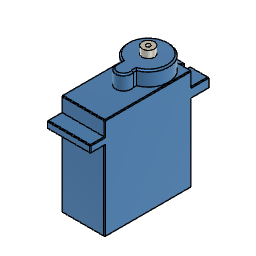
Servo Motor (Autodesk Fusion 360 design; units mm, degrees)
Autodesk Fusion 360 part; units mm, degrees
note: some values were not read from the file. Chosen so that the rebuilt part matches the saved one: a direction.
sketch "Sketch1" plane through (0, 0, 0) normal (1, 0, 0) x (0, 1, 0)
  line L0 (0, 0) -> (60, 0)
  line L1 (60, 0) -> (60, 70)
  line L2 (60, 70) -> (0, 70)
  line L3 (0, 70) -> (0, 0)
  line L4 (0, 50) -> (60, 50)
  dimension "d1" = 60
  dimension "d2" = 70
  constraint horizontal L0
  constraint vertical L1
  constraint horizontal L2
  constraint vertical L3
  constraint coincident L0.start L3.end
  constraint coincident L3 L4.start
  constraint perpendicular L3 L4
  constraint coincident L1 L4.end
  measures "d1" distance of L1.end L2.end
  measures "d2" vertical distance of L0.start L1.end
extrude "Extrude1" add sketch "Sketch1" along normal blind 30 makes body 1
sketch "Sketch2" plane through (0, 0, 70) normal (0, 0, 1) x (-1, 0, 0)
  line L0 (0, -60) -> (0, 0)
  line L1 (0, 0) -> (-30, 0)
  line L2 (-30, 0) -> (-30, -60)
  line L3 (-30, -60) -> (0, -60)
  circle A0 centre (-15, -45) radius 4.4943
  circle A1 centre (-15, -45) radius 1.0141
  line L4 (-10.0834, -31.5246) -> (-10.0834, -25)
  line L5 (-19.9166, -31.5246) -> (-19.9166, -25)
  arc A2 (-10.0834, -25) -> (-19.9166, -25) centre (-15, -25) ccw
  arc A3 (-19.9166, -31.5246) -> (-10.0834, -31.5246) centre (-15, -45) ccw
  dimension "d5" = 28.6886
  dimension "d6" = 8.9885
  dimension "d7" = 2.0283
  dimension "d8" = 9.8331
  constraint concentric A0 A3
  constraint concentric A0 A1
  constraint parallel L0 L4
  constraint parallel L4 L5
  constraint tangent L5 A2
  measures "d5" diameter of A3
  measures "d6" diameter of A0
  measures "d7" diameter of A1
  measures "d8" distance of L4.end L5.end
extrude "Extrude3" add sketch "Sketch2" along normal blind 15 contours A0 bodies 1
sketch "Sketch3" plane through (0, 60, 0) normal (0, 1, 0) x (-1, 0, 0)
  line L0 (0, 0) -> (0, 70)
  line L1 (0, 70) -> (-30, 70)
  line L2 (-30, 70) -> (-30, 0)
  line L3 (-30, 0) -> (0, 0)
  line L4 (-30, 60) -> (0, 60)
  line L5 (0, 60) -> (0, 53.1514)
  line L6 (0, 53.1514) -> (-30, 53.1514)
  line L7 (-30, 53.1514) -> (-30, 60)
  constraint horizontal L4
  constraint vertical L5
  constraint horizontal L6
  constraint vertical L7
  constraint coincident L0 L5.end
  constraint coincident L2 L4.start
extrude "Extrude4" add sketch "Sketch3" along normal blind 12 contours L0 L2 L4 L5 L6 L7 bodies 1
sketch "Sketch4" plane through (0, 0, 60) normal (0, 0, 1) x (-1, 0, 0)
  line L0 (0, -60) -> (-30, -60)
  line L1 (-30, -60) -> (-30, -72)
  line L2 (-30, -72) -> (0, -72)
  line L3 (0, -72) -> (0, -60)
  line L4 (-15, -72) -> (-17, -72)
  line L5 (-15, -72) -> (-13, -72)
  line L6 (-13, -72) -> (-13, -70)
  line L7 (-17, -72) -> (-17, -70)
  arc A0 (-13, -70) -> (-17, -70) centre (-15, -67) ccw
  dimension "d16" = 7.2111
  constraint midpoint L2 L4.start
  constraint coincident L2 L4.end
  constraint parallel L2 L4
  constraint coincident L2 L5.end
  constraint perpendicular L2 L6
  constraint perpendicular L2 L7
  measures "d16" diameter of A0
extrude "Extrude5" cut sketch "Sketch4" against normal through all contours L2 L4 L5 L6 L7 A0 bodies 1
chamfer "Chamfer2" distance 0.5 angle 45 7 edges at (15, 63.3944, 60) (0, 66, 60) (30, 66, 60) (23.5, 72, 60) (6.5, 72, 60) (6.5, 72, 53.1514) (23.5, 72, 53.1514) on bodies 1
chamfer "Chamfer3" distance 0.5 angle 45 7 edges at (0, 65.75, 53.1514) (30, 65.75, 53.1514) (15, 63.3944, 53.1514) (17, 70.75, 53.1514) (13, 70.75, 53.1514) (13, 71.0427, 60) (17, 71.0427, 60) on bodies 1
sketch "Sketch5" plane through (0, 0, 0) normal (0, -1, 0) x (1, 0, 0)
  line L0 (0, 70) -> (0, 0)
  line L1 (0, 0) -> (30, 0)
  line L2 (30, 0) -> (30, 70)
  line L3 (30, 70) -> (0, 70)
  line L4 (0, 60) -> (30, 60)
  line L5 (30, 60) -> (30, 55)
  line L6 (30, 55) -> (0, 55)
  line L7 (0, 55) -> (0, 60)
  constraint horizontal L4
  constraint vertical L5
  constraint horizontal L6
  constraint vertical L7
  constraint coincident L2 L5.end
  constraint coincident L0 L4.start
extrude "Extrude6" add sketch "Sketch5" along normal blind 10 contours L0 L2 L4 L5 L6 L7 bodies 1
chamfer "Chamfer4" distance 0.5 angle 45 8 edges at (30, 30, 70) (30, 60, 26.8257) (30, 0, 27.5) (30, -5, 55) (30, -5, 60) (30, 60, 64.75) (30, 0, 65) (30, 30, 0) on bodies 1
chamfer "Chamfer5" distance 0.5 angle 45 14 edges at (0, 30, 70) (0, 60, 64.75) (0, 60, 26.8257) (0, 0, 65) (0, 0, 27.5) (0, -5, 55) (0, -5, 60) (14.75, -10, 55) (14.75, -10, 60) (30, -10, 57.5) (0, -10, 57.5) (0, 30, 0) (14.75, 0, 0) (29.5, 0, 27.5) on bodies 1
chamfer "Chamfer6" distance 0.5 angle 45 2 edges at (15, 60, 70) (15, 0, 70) on bodies 1
chamfer "Chamfer7" distance 0.5 angle 45 1 edges at (15, 60, 0) on bodies 1
delete_face "DeleteFace1" 1 faces at (10.5281, 45.4475, 80) on bodies 1
sketch "Sketch6" plane through (0, 0, 70) normal (0, 0, 1) x (-1, 0, 0)
  line L0 (-0.5, -0.5) -> (-29.5, -0.5)
  line L1 (-29.5, -0.5) -> (-29.5, -59.5)
  line L2 (-29.5, -59.5) -> (-0.5, -59.5)
  line L3 (-0.5, -59.5) -> (-0.5, -0.5)
  circle A0 centre (-15, -45) radius 4.2399
  circle A1 centre (-15, -45) radius 1.4688
  line L4 (-9.8947, -31.8115) -> (-9.8947, -27.8115)
  line L5 (-20.1053, -31.8115) -> (-20.1053, -27.8115)
  arc A2 (-9.8947, -28.7128) -> (-20.1053, -29.5551) centre (-15.1091, -27.8115) ccw
  arc A3 (-20.1053, -31.8115) -> (-9.8947, -31.8115) centre (-15, -45) ccw
  dimension "d26" = 28.2843
  dimension "d27" = 8.4797
  dimension "d28" = 2.9377
  dimension "d29" = 4
  dimension "d30" = 10.5834
  constraint concentric A0 A3
  constraint concentric A1 A3
  constraint vertical L4
  constraint parallel L4 L5
  constraint coincident L4 A2.start
  constraint coincident L5 A2.end
  measures "d26" diameter of A3
  measures "d27" diameter of A0
  measures "d28" diameter of A1
  measures "d29" distance of L4.start L4.end
  measures "d30" diameter of A2
extrude "Extrude7" add sketch "Sketch6" along normal blind 10 contours L4 L5 A2 A3 bodies 1
extrude "Extrude8" add sketch "Sketch6" along normal blind 15 separate body contours A0 makes body 2
chamfer "Chamfer8" distance 1 angle 45 4 edges at (15, 59.1421, 80) (15.5441, 22.5377, 80) (9.8947, 30.2622, 80) (20.1053, 30.6833, 80) on bodies 1
